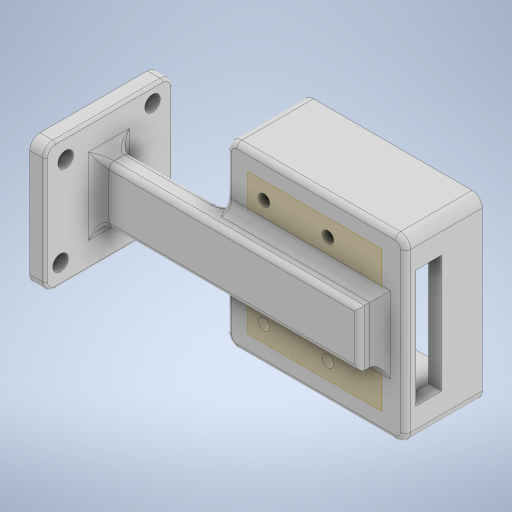
# Autodesk Inventor part: cover_part
Saved by Autodesk Inventor 2024 (Build 280153000, 153)
## iProperties
Created: 2024-05-03
Part Number: cover_part
Material: Generic
Document SubType Name: Modeling
Designer: Pintu
Density: 1 g/cm^3
Appearance: Default
Author: Pintu
Autodesk Inventor part; units mm, degrees
ref_plane "YZ Plane" through (0, 0, 0) normal (1, 0, 0) x (0, 1, 0)
ref_plane "XZ Plane" through (0, 0, 0) normal (0, 1, 0) x (-1, 0, 0)
ref_plane "XY Plane" through (0, 0, 0) normal (0, 0, 1) x (1, 0, 0)
ref_plane "Work Plane1" through (0.2337, 0, 5.0432) normal (0, 0, 1) x (1, 0, 0)
sketch "Sketch1" plane through (0.2337, 0, 5.0432) normal (0, 0, 1) x (1, 0, 0)
  line L0 (-17.5, -17.5) -> (17.5, -17.5)
  line L1 (17.5, -17.5) -> (17.5, 17.5)
  line L2 (17.5, 17.5) -> (-17.5, 17.5)
  line L3 (-17.5, 17.5) -> (-17.5, -17.5)
  line L4 (-17.5, -17.5) -> (17.5, 17.5) construction
  line L5 (17.5, -17.5) -> (-17.5, 17.5) construction
  line L6 (-15, -15) -> (15, -15)
  line L7 (15, -15) -> (15, 15)
  line L8 (15, 15) -> (-15, 15)
  line L9 (-15, 15) -> (-15, -15)
  point P0 (-0.2337, 0)
  point P1 (0, 0)
  dimension "d0" = 35
  dimension "d1" = 35
  dimension "d2" = 2.5
  constraints: 20 end point, 4 parallel, 2 midpoint, 2 perpendicular, 1 horizontal, 3 other
  measures "d0" distance of L2.end L1.end
  measures "d1" distance of L1.end L0.end
  measures "d2" distance between parallel lines of L3 L9
extrude "Extrusion1" add sketch "Sketch1" against normal blind 12
extrude "Extrusion2" add sketch "Sketch1" against normal blind 2 contours L9 L8 L7 L6
sketch "Sketch2" plane through (0.2337, 0, 3.0432) normal (0, 0, -1) x (-1, 0, 0)
  circle A0 centre (10.1647, 10.5) radius 1.1 projected
  circle A1 centre (-2.3353, 10.5) radius 1.1 projected
  line L0 (-15, -15) -> (-15, 15) projected
  line L1 (15, -15) -> (-15, -15) projected
  line L2 (15, 15) -> (15, -15) projected
  line L3 (-15, 15) -> (15, 15) projected
  circle A2 centre (-2.3353, -10.5) radius 1.1 projected
  circle A3 centre (10.1647, -10.5) radius 1.1 projected
  circle A4 centre (10.1647, -10.5) radius 2.35
  circle A5 centre (-2.3353, -10.5) radius 2.35
  circle A6 centre (-2.3353, 10.5) radius 2.35
  circle A7 centre (10.1647, 10.5) radius 2.35
  point P0 (0.2337, 0)
  dimension "d7" = 1.25
  dimension "d8" = 1.25
  dimension "d9" = 1.25
  dimension "d10" = 1.25
  constraints: 4 centre point
  measures "d7" radial gap between concentric circles of A3 A4
  measures "d8" radial gap between concentric circles of A2 A5
  measures "d9" radial gap between concentric circles of A1 A6
  measures "d10" radial gap between concentric circles of A0 A7
extrude "Extrusion3" add sketch "Sketch2" along normal blind 3 contours A4 | A5 | A6 | A7
fillet "Fillet1" radius 2 8 edges at (-14.7663, 15, -1.9568) (-17.2663, 17.5, -0.9568) (-14.7663, -15, -1.9568) (-17.2663, -17.5, -0.9568) (15.2337, -15, -1.9568) (17.7337, -17.5, -0.9568) (15.2337, 15, -1.9568) (17.7337, 17.5, -0.9568)
sketch "Sketch3" plane through (0.2337, 0, 3.0432) normal (0, 0, -1) x (-1, 0, 0)
  circle A0 centre (10.1647, -10.5) radius 1.1 projected
  circle A1 centre (-2.3353, -10.5) radius 1.1 projected
  circle A2 centre (-2.3353, 10.5) radius 1.1 projected
  circle A3 centre (10.1647, 10.5) radius 1.1 projected
  point P0 (0.2337, 0)
extrude "Extrusion4" cut sketch "Sketch3" against normal blind 4
sketch "Sketch5" plane through (15.2337, -13, -6.9568) normal (-1, 0, 0) x (0, 0, 1)
  line L0 (10, 0) -> (10, 26) projected
  line L1 (10, 24.5) -> (5, 24.5)
  line L2 (5, 24.5) -> (5, 1.5)
  line L3 (5, 1.5) -> (10, 1.5)
  line L4 (10, 1.5) -> (10, 24.5)
  line L5 (12, -4.5) -> (0, -4.5) projected
  point P0 (6.9568, 13)
  point P1 (7.5, 1.5)
  point P2 (10, 1.5)
  dimension "d22" = 5
  dimension "d23" = 23
  dimension "d24" = 6
  constraints: 8 end point, 2 parallel, 1 horizontal, 1 midpoint, 1 perpendicular, 1 point on line
  measures "d22" distance of L3.end L2.end
  measures "d23" distance of L2.end L1.end
  measures "d24" distance from line of L5 point (7.5, 1.5)
extrude "Extrusion6" cut sketch "Sketch5" against normal blind 110.5
sketch "Sketch6" plane through (-14.7663, -13, -6.9568) normal (1, 0, 0) x (0, 0, -1)
  line L0 (-10, 1.5) -> (-10, 24.5) projected
  line L1 (-10, 24.5) -> (-5, 24.5) projected
  line L2 (-5, 24.5) -> (-5, 1.5) projected
  line L3 (-5, 1.5) -> (-10, 1.5) projected
  line L4 (-12, 28.5) -> (0, 28.5) projected
  line L5 (-12, -2.5) -> (-12, 28.5) projected
  line L6 (0, -2.5) -> (-12, -2.5) projected
  line L7 (0, 28.5) -> (0, -2.5) projected
  point P0 (-6.9568, 13)
extrude "Extrusion7" cut sketch "Sketch6" against normal blind 110.5 contours L0 L1 L2 L3
sketch "Sketch7" plane through (0.2337, 0, 5.0432) normal (0, 0, 1) x (1, 0, 0)
  line L0 (12.5, 5.5) -> (-41.5, 5.5)
  line L1 (-41.5, 5.5) -> (-41.5, -5.5)
  line L2 (-41.5, -5.5) -> (12.5, -5.5)
  line L3 (12.5, -5.5) -> (12.5, 5.5)
  line L4 (-15.5, -17.5) -> (15.5, -17.5) projected
  line L5 (15.5, 17.5) -> (-15.5, 17.5) projected
  line L6 (17.5, -15.5) -> (17.5, 15.5) projected
  line L7 (-17.5, 15.5) -> (-17.5, -15.5) projected
  point P0 (-0.2337, 0)
  dimension "d31" = 12
  dimension "d32" = 12
  dimension "d33" = 5
  dimension "d34" = 24
  constraints: 8 end point, 2 parallel, 1 horizontal, 1 perpendicular
  measures "d31" distance between parallel lines of L4 L2
  measures "d32" distance between parallel lines of L5 L0
  measures "d33" distance between parallel lines of L6 L3
  measures "d34" distance between parallel lines of L7 L1
extrude "Extrusion8" add sketch "Sketch7" along normal blind 4
sketch "Sketch8" plane through (-41.2663, -5.5, 5.0432) normal (-1, 0, 0) x (0, 0, 1)
  line L0 (0, 11) -> (0, 0) projected
  line L1 (0, 0) -> (4, 0) projected
  line L2 (4, 11) -> (4, 0) projected
  line L3 (0, 11) -> (4, 11) projected
  line L4 (-10.5, -7) -> (14.5, -7)
  line L5 (14.5, -7) -> (14.5, 18)
  line L6 (14.5, 18) -> (-10.5, 18)
  line L7 (-10.5, 18) -> (-10.5, -7)
  line L8 (-10.5, -7) -> (14.5, 18) construction
  line L9 (14.5, -7) -> (-10.5, 18) construction
  point P0 (-5.0432, 5.5)
  point P1 (2, 5.5)
  dimension "d35" = 25
  dimension "d36" = 25
  constraints: 12 end point, 2 midpoint, 2 parallel, 1 horizontal, 1 perpendicular
  measures "d35" distance of L6.end L5.end
  measures "d36" distance of L5.end L4.end
extrude "Extrusion9" add sketch "Sketch8" against normal blind 3
sketch "Sketch9" plane through (-38.2663, -5.5, 5.0432) normal (1, 0, 0) x (0, 0, -1)
  line L0 (-14.5, 18) -> (-14.5, -7) projected
  line L1 (10.5, 18) -> (-14.5, 18) projected
  point P0 (5.0432, 5.5)
  point P1 (-10.5, 14)
  dimension "d39" = 4
  dimension "d40" = 4
  measures "d39" distance from line of L0 point (-10.5, 14)
  measures "d40" distance from line of L1 point (-10.5, 14)
hole "Hole1" at (-38.2663, 8.5, 15.5432) direction (-1, 0, 0) diameter 3 depth 25 tip angle 118
sketch "Sketch10" plane through (-38.2663, -5.5, 5.0432) normal (1, 0, 0) x (0, 0, -1)
  line L0 (-14.5, -7) -> (10.5, -7) projected
  line L1 (-14.5, 18) -> (-14.5, -7) projected
  point P0 (5.0432, 5.5)
  point P1 (-11.5, -3)
  dimension "d48" = 4
  dimension "d49" = 3
  measures "d48" distance from line of L0 point (-11.5, -3)
  measures "d49" distance from line of L1 point (-11.5, -3)
hole "Hole2" at (-38.2663, -8.5, 16.5432) direction (-1, 0, 0) diameter 3 depth 25 tip angle 118
sketch "Sketch11" plane through (-38.2663, -5.5, 5.0432) normal (1, 0, 0) x (0, 0, -1)
  line L0 (10.5, -7) -> (10.5, 18) projected
  line L1 (-14.5, -7) -> (10.5, -7) projected
  point P0 (5.0432, 5.5)
  point P1 (6.5, -3)
  dimension "d57" = 4
  dimension "d58" = 4
  measures "d57" distance from line of L0 point (6.5, -3)
  measures "d58" distance from line of L1 point (6.5, -3)
hole "Hole3" at (-38.2663, -8.5, -1.4568) direction (-1, 0, 0) diameter 3 depth 25 tip angle 118
sketch "Sketch12" plane through (-38.2663, -5.5, 5.0432) normal (1, 0, 0) x (0, 0, -1)
  line L0 (10.5, -7) -> (10.5, 18) projected
  line L1 (10.5, 18) -> (-14.5, 18) projected
  point P0 (5.0432, 5.5)
  point P1 (6.5, 15)
  dimension "d66" = 4
  dimension "d67" = 3
  measures "d66" distance from line of L0 point (6.5, 15)
  measures "d67" distance from line of L1 point (6.5, 15)
hole "Hole4" at (-38.2663, 9.5, -1.4568) direction (-1, 0, 0) diameter 3 depth 25 tip angle 118
fillet "Fillet2" radius 2 8 edges at (-39.7663, -12.5, -5.4568) (-39.7663, 12.5, -5.4568) (-39.7663, 12.5, 19.5432) (-39.7663, -12.5, 19.5432) (-38.2663, 0, 9.0432) (-38.2663, 0, 5.0432) (-38.2663, 5.5, 7.0432) (-38.2663, -5.5, 7.0432)
fillet "Fillet3" radius 2 3 edges at (-2.2663, -5.5, 5.0432) (-2.2663, 5.5, 5.0432) (12.7337, 0, 5.0432)
fillet "Fillet4" radius 1 5 edges at (-37.6805, 6.0858, 9.629) (-11.7663, 5.5, 9.0432) (-37.6805, -6.0858, 9.629) (-11.7663, -5.5, 9.0432) (12.7337, 0, 9.0432)
fillet "Fillet5" radius 1 11 edges at (-16.6805, 16.9142, 5.0432) (-17.2663, 11.5, 5.0432) (-17.2663, 6.0858, 5.629) (17.1479, 16.9142, 5.0432) (17.7337, 0, 5.0432) (17.1479, -16.9142, 5.0432) (0.2337, -17.5, 5.0432) (-16.6805, -16.9142, 5.0432) (-17.2663, -11.5, 5.0432) (-17.2663, -6.0858, 5.629) (0.2337, 17.5, 5.0432)
fillet "Fillet7" radius 2 3 edges at (-17.2625, -5.3819, 5.0432) (-17.2625, 5.3819, 5.0432) (-17.2663, 0, 5.0432)
fillet "Fillet8" radius 1 6 edges at (-37.6805, 6.0858, 4.4574) (-17.8521, 5.5, 4.4574) (-27.7663, 5.5, 5.0432) (-17.8521, -5.5, 4.4574) (-37.6805, -6.0858, 4.4574) (-27.7663, -5.5, 5.0432)
fillet "Fillet9" radius 0.5 8 edges at (-38.2663, 11.9142, 18.9574) (-38.2663, 0, 19.5432) (-38.2663, -11.9142, 18.9574) (-38.2663, -12.5, 7.0432) (-38.2663, -11.9142, -4.871) (-38.2663, 0, -5.4568) (-38.2663, 11.9142, -4.871) (-38.2663, 12.5, 7.0432)
fillet "Fillet11" radius 0.5 10 edges at (14.6479, -14.4142, 3.0432) (15.2337, -12.25, 3.0432) (-14.1805, -14.4142, 3.0432) (-14.7663, -12.25, 3.0432) (0.2337, -15, 3.0432) (15.2337, 12.25, 3.0432) (0.2337, 15, 3.0432) (-14.1805, 14.4142, 3.0432) (-14.7663, 12.25, 3.0432) (14.6479, 14.4142, 3.0432)
sketch "Sketch13" plane through (0.2337, 0, -6.9568) normal (0, 0, -1) x (-1, 0, 0)
  arc A0 (-15.5, 17.5) -> (-17.5, 15.5) centre (-15.5, 15.5) ccw projected
  line L0 (-17.5, 15.5) -> (-17.5, -15.5) projected
  arc A1 (-17.5, -15.5) -> (-15.5, -17.5) centre (-15.5, -15.5) ccw projected
  line L1 (-15.5, -17.5) -> (15.5, -17.5) projected
  arc A2 (15.5, -17.5) -> (17.5, -15.5) centre (15.5, -15.5) ccw projected
  line L2 (17.5, -15.5) -> (17.5, 15.5) projected
  arc A3 (17.5, 15.5) -> (15.5, 17.5) centre (15.5, 15.5) ccw projected
  line L3 (15.5, 17.5) -> (-15.5, 17.5) projected
  line L4 (15, 13) -> (15, -13) projected
  arc A4 (13, -15) -> (15, -13) centre (13, -13) ccw projected
  line L5 (13, -15) -> (-13, -15) projected
  arc A5 (-15, -13) -> (-13, -15) centre (-13, -13) ccw projected
  line L6 (-15, -13) -> (-15, 13) projected
  arc A6 (-13, 15) -> (-15, 13) centre (-13, 13) ccw projected
  line L7 (-13, 15) -> (13, 15) projected
  arc A7 (15, 13) -> (13, 15) centre (13, 13) ccw projected
  point P0 (0.2337, 0)
extrude "Extrusion10" add sketch "Sketch13" along normal blind 3
body "Solid1"
